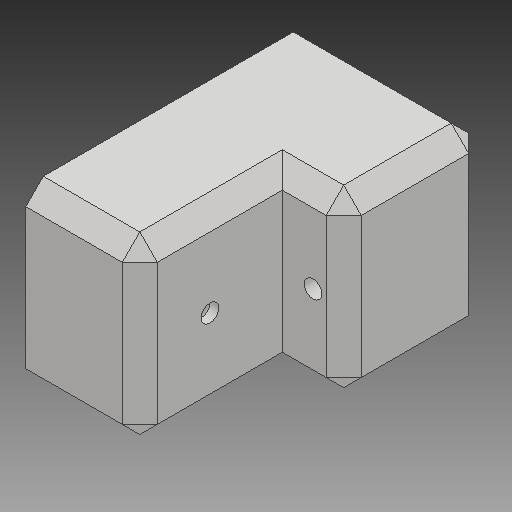
# Autodesk Inventor part: 1
Saved by Autodesk Inventor 2021 (Build 250183000, 183)
## iProperties
Company: HTBLA Kaindorf
RuleStatus: InUse
Created: 2021-12-20
Part Number: 1
Project: Default
Material: Generisch
Document SubType Name: Modeling
Designer: LFL
Density: 1 g/cm^3
Appearance: Vorgabe
Mass: 7.03683 g
Surface Area: 40.0099 cm^2
Volume: 7.03683 cm^3
Stock Number: Nukleatordüse
AfterDocNew0: iProperties-Editor_aufrufen
Author: CADKustos
Autodesk Inventor part; units mm, degrees
ref_plane "YZ Plane" through (0, 0, 0) normal (1, 0, 0) x (0, 1, 0)
ref_plane "XZ Plane" through (0, 0, 0) normal (0, 1, 0) x (-1, 0, 0)
ref_plane "XY Plane" through (0, 0, 0) normal (0, 0, 1) x (1, 0, 0)
sketch "Skizze3" plane through (0, 0, 0) normal (0, 0, 1) x (1, 0, 0)
  line L0 (-22.75, 0) -> (22.75, 0) projected
  line L1 (0, -17) -> (0, 11) projected
  line L2 (-16.25, 7) -> (0, 7)
  line L3 (16.25, 0) -> (16.25, -13)
  line L4 (16.25, -13) -> (-16.25, -13)
  line L5 (-16.25, -13) -> (-16.25, 7)
  line L6 (0, 7) -> (0, 0)
  line L7 (16.25, 0) -> (0, 0)
  point P0 (16.25, 0)
  point P1 (0, 7)
  dimension "d4" = 20
  dimension "d5" = 32.5
  dimension "d41" = 7
  constraints: 12 end point, 2 parallel, 2 perpendicular, 1 collinear, 1 horizontal, 1 other
  measures "d4" distance between parallel lines of L2 L4
  measures "d5" distance between parallel lines of L3 L5
  measures "d41" distance between parallel lines of L0 L2
extrude "Extrusion3" add sketch "Skizze3" along normal blind 20
sketch "Skizze6" plane through (0, 0, 0) normal (0, 1, 0) x (1, 0, 0)
  line L0 (16.25, 0) -> (0, 0) projected
  line L1 (16.25, 0) -> (16.25, -20) projected
  circle A0 centre (8.25, -10) radius 1
  dimension "d21" = 10
  dimension "d22" = 8
  dimension "d23" = 2
  constraints: 1 centre point, 1 coincident
  measures "d21" distance from line of L0 point (8.25, -10)
  measures "d22" distance from line of point (8.25, -10) L1
  measures "d23" diameter of A0
extrude "Extrusion6" cut sketch "Skizze6" against normal blind 3
sketch "Skizze7" plane through (0, 0, 0) normal (1, 0, 0) x (0, 0, -1)
  line L0 (0, 0) -> (0, 7) projected
  line L1 (0, 7) -> (-20, 7) projected
  circle A0 centre (-10, 3.5) radius 1
  dimension "d26" = 10
  dimension "d27" = 3.5
  dimension "d28" = 2
  constraints: 1 centre point, 1 coincident
  measures "d26" distance from line of point (-10, 3.5) L0
  measures "d27" distance from line of L1 point (-10, 3.5)
  measures "d28" diameter of A0
extrude "Extrusion7" cut sketch "Skizze7" against normal blind 10
chamfer "Fase4" distance 2 angle 45 13 edges at (-8.125, 7, 20) (-16.25, -3, 20) (-16.25, 7, 10) (-16.25, -3, 0) (-8.125, 7, 0) (0, 7, 10) (8.125, 0, 0) (8.125, 0, 20) (16.25, 0, 10) (16.25, -6.5, 0) (16.25, -6.5, 20) (0, 3.5, 20) (0, 3.5, 0)
sketch "Skizze9" plane through (-14.25, -13, 0) normal (0, -1, 0) x (1, 0, 0)
  circle A0 centre (22.5, 10) radius 1 projected
  line L0 (-2, 2) -> (-2, 18) projected
  point P0 (14.25, 0)
  constraints: 1 coincident
hole "Bohrung1" at (8.25, -13, 10) direction (0, 1, 0) diameter 11.445 depth 12 thread size "G13.157x1.337" designation "G 1/4" standard "ISO Pipe Threads"
sketch "Skizze10" plane through (-14.25, -13, 0) normal (0, -1, 0) x (1, 0, 0)
  line L0 (0, 0) -> (28.5, 0) projected
  line L1 (-2, 2) -> (-2, 18) projected
  point P0 (14.25, 0)
  point P1 (6, 10)
  dimension "d53" = 10
  dimension "d54" = 8
  measures "d53" distance from line of point (6, 10) L0
  measures "d54" distance from line of point (6, 10) L1
hole "Bohrung2" at (-8.25, -13, 10) direction (0, 1, 0) diameter 11.445 depth 18 thread size "G13.157x1.337" designation "G 1/4" standard "ISO Pipe Threads"
